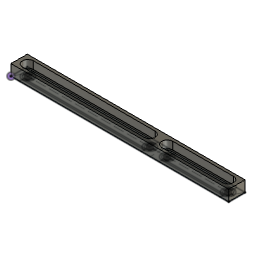
n_ext_1 v1 (Autodesk Fusion 360 design; units mm, degrees)
Autodesk Fusion 360 part; units mm, degrees
sketch "Sketch1" plane through (0, 0, 0) normal (0, 0, 1) x (1, 0, 0)
  line L0 (0, 0) -> (200, 0)
  line L1 (200, 0) -> (200, 15)
  line L2 (200, 15) -> (0, 15)
  line L3 (0, 15) -> (0, 0)
  line L4 (192, 15) -> (192, 0) construction
  line L5 (8, 15) -> (8, 0) construction
  line L6 (200, 15) -> (192, 0) construction
  line L7 (192, 15) -> (200, 0) construction
  line L8 (0, 0) -> (8, 15) construction
  line L9 (0, 15) -> (8, 0) construction
  line L10 (4, 7.5) -> (196, 7.5) construction
  circle A0 centre (8, 7.5) radius 5
  circle A1 centre (192, 7.5) radius 5
  line L11 (128, 15) -> (128, 0) construction
  line L12 (136, 15) -> (136, 0) construction
  line L13 (120, 15) -> (120, 0) construction
  circle A2 centre (136, 7.5) radius 5
  circle A3 centre (120, 7.5) radius 5
  circle A4 centre (8, 7.5) radius 3.5
  circle A5 centre (120, 7.5) radius 3.5
  circle A6 centre (136, 7.5) radius 3.5
  circle A7 centre (192, 7.5) radius 3.5
  line L14 (8, 12.5) -> (120, 12.5)
  line L15 (8, 11) -> (120, 11)
  line L16 (8, 4) -> (120, 4)
  line L17 (8, 2.5) -> (120, 2.5)
  line L18 (136, 12.5) -> (192, 12.5)
  line L19 (136, 11) -> (192, 11)
  line L20 (136, 4) -> (192, 4)
  line L21 (136, 2.5) -> (192, 2.5)
  dimension "d1" = 200
  dimension "d2" = 15
  dimension "d3" = 8
  dimension "d4" = 8
  dimension "d5" = 10
  dimension "d6" = 10
  dimension "d7" = 64
  dimension "d8" = 8
  dimension "d9" = 8
  dimension "d10" = 10
  dimension "d11" = 10
  dimension "d12" = 7
  dimension "d13" = 7
  dimension "d14" = 7
  dimension "d15" = 7
  constraint horizontal L0
  constraint vertical L1
  constraint horizontal L2
  constraint vertical L3
  constraint coincident L0.start L3.end
  constraint coincident L2 L4.start
  constraint coincident L0 L4.end
  constraint perpendicular L0 L4
  constraint coincident L2 L5.start
  constraint coincident L0 L5.end
  constraint perpendicular L0 L5
  constraint midpoint L8 L10.start
  constraint midpoint L6 L10.end
  constraint midpoint L5 A0.centre
  constraint midpoint L4 A1.centre
  constraint coincident L2 L11.start
  constraint coincident L0 L11.end
  constraint perpendicular L0 L11
  constraint coincident L2 L12.start
  constraint coincident L0 L12.end
  constraint perpendicular L0 L12
  constraint coincident L2 L13.start
  constraint coincident L0 L13.end
  constraint perpendicular L0 L13
  constraint midpoint L12 A2.centre
  constraint midpoint L13 A3.centre
  constraint concentric A0 A4
  constraint concentric A3 A5
  constraint concentric A2 A6
  constraint concentric A1 A7
  constraint coincident A0 L14.start
  constraint coincident L5 L14.start
  constraint coincident A3 L14.end
  constraint coincident L13 L14.end
  constraint coincident L5 L15.start
  constraint coincident A4 L15.start
  constraint coincident L13 L15.end
  constraint coincident A5 L15.end
  constraint coincident L5 L16.start
  constraint coincident A4 L16.start
  constraint coincident L13 L16.end
  constraint coincident A5 L16.end
  constraint coincident L5 L17.start
  constraint coincident A0 L17.start
  constraint coincident A3 L17.end
  constraint coincident L13 L17.end
  constraint coincident A2 L18.start
  constraint coincident L12 L18.start
  constraint coincident A1 L18.end
  constraint coincident L4 L18.end
  constraint coincident L12 L19.start
  constraint coincident A6 L19.start
  constraint coincident A7 L19.end
  constraint coincident L4 L19.end
  constraint coincident L12 L20.start
  constraint coincident A6 L20.start
  constraint coincident A7 L20.end
  constraint coincident L4 L20.end
  constraint coincident A2 L21.start
  constraint coincident L12 L21.start
  constraint coincident A1 L21.end
  constraint coincident L4 L21.end
  measures "d1" distance of L0.start L0.end
  measures "d2" distance of L0.start L2.end
  measures "d3" distance of L3 L5
  measures "d4" distance of L1 L4
  measures "d5" diameter of A0
  measures "d6" diameter of A1
  measures "d7" distance of L4 L11
  measures "d8" distance of L11 L12
  measures "d9" distance of L11 L13
  measures "d10" diameter of A2
  measures "d11" diameter of A3
  measures "d12" diameter of A4
  measures "d13" diameter of A5
  measures "d14" diameter of A6
  measures "d15" diameter of A7
extrude "Extrude1" add sketch "Sketch1" along normal blind 10 makes body 1
extrude "Extrude2" add sketch "Sketch1" along normal blind 3 separate body contours A0 A4 L15 L16 | A0 A3 L14 L15 | A0 A3 L16 L17 | A3 A5 L15 L16 | A1 A7 L19 L20 | A1 A2 L18 L19 | A1 A2 L20 L21 | A2 A6 L19 L20 picked at (6.4417, 11.7091) picked at (124.4712, 7.0968) picked at (193.6466, 3.3236) picked at (133.8318, 11.4298) makes body 2 at (82.6667, 11.5, 3) makes body 3 at (154.6667, 3.5, 0)
